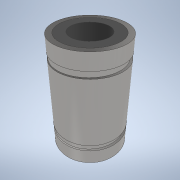
# Autodesk Inventor part: Линейный подшипник
Saved by Autodesk Inventor 2021.1 (Build 251245010, 245A)
## iProperties
Created: 2022-01-10
Part Number: Линейный подшипник
Material: Типовые
Document SubType Name: Modeling
Designer: Andrew
Density: 1 g/cm^3
Appearance: По умолчанию
Author: Andrew
Autodesk Inventor part; units mm, degrees
ref_plane "YZ Plane" through (0, 0, 0) normal (1, 0, 0) x (0, 1, 0)
ref_plane "XZ Plane" through (0, 0, 0) normal (0, 1, 0) x (-1, 0, 0)
ref_plane "XY Plane" through (0, 0, 0) normal (0, 0, 1) x (1, 0, 0)
sketch "Эскиз1" plane through (0, 0, 0) normal (0, 1, 0) x (-1, 0, 0)
  circle A0 centre (-0.2416, 0) radius 7.5
  circle A1 centre (-0.2416, 0) radius 6.3
  point P0 (0, 0)
  dimension "d0" = 15
  dimension "d2" = 12.6
  constraints: 2 centre point
  measures "d0" diameter of A0
  measures "d2" diameter of A1
extrude "Выдавливание1" add sketch "Эскиз1" along normal blind 24
sketch "Эскиз2" plane through (0.2416, 24, 0) normal (0, 1, 0) x (1, 0, 0)
  circle A0 centre (0, 0) radius 6.3 projected
  circle A1 centre (0, 0) radius 4
  circle A2 centre (0, 0) radius 6.3
  point P0 (-0.2416, 0)
  dimension "d7" = 8
  dimension "d8" = 12.6
  constraints: 2 centre point, 2 coincident
  measures "d7" diameter of A1
  measures "d8" diameter of A2
extrude "Выдавливание2" add sketch "Эскиз2" against normal blind 24 separate body
sketch "Эскиз3" plane through (0, 0, 0) normal (1, 0, 0) x (0, 1, 0)
  line L0 (20.7, 9.5) -> (19.3, 9.5)
  line L1 (19.3, 9.5) -> (19.3, 7.2)
  line L2 (19.3, 7.2) -> (20.7, 7.2)
  line L3 (20.7, 7.2) -> (20.7, 9.5)
  line L4 (4.7, 9.5) -> (3.3, 9.5)
  line L5 (3.3, 9.5) -> (3.3, 7.2)
  line L6 (3.3, 7.2) -> (4.7, 7.2)
  line L7 (4.7, 7.2) -> (4.7, 9.5)
  line L8 (24, -7.5) -> (24, 7.5) projected
  line L9 (0, -7.5) -> (0, 7.5) projected
  line L10 (24, 7.5) -> (0, 7.5) construction
  line L11 (-4.8, 0) -> (28.8, 0) projected
  point P0 (0, 0)
  dimension "d11" = 1.4
  dimension "d12" = 1.4
  dimension "d13" = 3.3
  dimension "d14" = 3.3
  dimension "d15" = 0.3
  dimension "d16" = 2
  constraints: 18 end point, 4 parallel, 3 horizontal, 2 collinear, 2 perpendicular
  measures "d11" distance between parallel lines of L3 L1
  measures "d12" distance between parallel lines of L7 L5
  measures "d13" distance between parallel lines of L3 L8
  measures "d14" distance between parallel lines of L9 L5
  measures "d15" distance between parallel lines of L10 L2
  measures "d16" distance between parallel lines of L0 L10
revolve "Вращение1" cut sketch "Эскиз3" angle 360 about axis through (0, -10, 0) along (0, 1, 0) bodies 1
equation "\"d12\" = d11"
